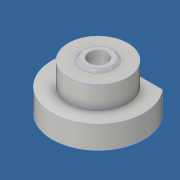
# Autodesk Inventor part: Belt_T_Spacer
Saved by Autodesk Inventor 2016 SP1 (Build 200210100, 210)
## iProperties
Created: 2015-09-20
Part Number: Belt_T_Spacer
Material: Aluminium 6061
Document SubType Name: Modeling
Designer: 4ndreas
Density: 2.7 g/cm^3
Appearance: Aluminium - flach
Mass: 5.22317 g
Surface Area: 11.7355 cm^2
Volume: 1.93451 cm^3
Author: 4ndreas
Autodesk Inventor part; units mm, degrees
ref_plane "YZ Plane" through (0, 0, 0) normal (1, 0, 0) x (0, 1, 0)
ref_plane "XZ Plane" through (0, 0, 0) normal (0, 1, 0) x (-1, 0, 0)
ref_plane "XY Plane" through (0, 0, 0) normal (0, 0, 1) x (1, 0, 0)
sketch "Skizze1" plane through (0, 0, 0) normal (0, 0, 1) x (1, 0, 0)
  circle A0 centre (0, 0) radius 10
  dimension "d0" = 20
  constraints: 1 centre point, 1 coincident
  measures "d0" diameter of A0
extrude "Extrusion1" add sketch "Skizze1" along normal blind 5
sketch "Skizze2" plane through (0, 0, 5) normal (0, 0, 1) x (1, 0, 0)
  circle A0 centre (0, 0) radius 6.5
  dimension "d3" = 13
  constraints: 1 centre point, 1 coincident
  measures "d3" diameter of A0
extrude "Extrusion2" add sketch "Skizze2" along normal blind 5
sketch "Skizze3" plane through (0, 0, 5) normal (0, 0, 1) x (1, 0, 0)
  circle A0 centre (0, 0) radius 6.5 projected
  circle A1 centre (0, 0) radius 10 projected
  line L0 (-7.5993, 6.5) -> (7.5993, 6.5)
  constraints: 2 end point, 2 point on circle, 1 horizontal, 1 tangent
extrude "Extrusion3" cut sketch "Skizze3" against normal through all contours L0 A1 picked at (4.4606, 7.0529)
sketch "Skizze4" plane through (0, 0, 10) normal (0, 0, 1) x (1, 0, 0)
  circle A0 centre (0, 0) radius 3
  dimension "d8" = 6
  constraints: 1 centre point, 1 coincident
  measures "d8" diameter of A0
extrude "Extrusion4" add sketch "Skizze4" along normal blind 0.5
sketch "Skizze5" plane through (0, 0, 10.5) normal (0, 0, 1) x (1, 0, 0)
  point P0 (0, 0)
hole "Bohrung1" at (0, 0, 10.5) direction (0, 0, -1) diameter 4 end through all
chamfer "Fase1" distance 0.5 angle 45 1 edges at (-3, 0, 10)
